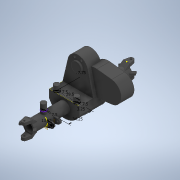
# Autodesk Inventor part: RCT-P004_front_rear_axle_simplified
Saved by Autodesk Inventor 2020 (Build 240168000, 168)
## iProperties
Created: 2019-11-14
Part Number: RCT-P004_front_rear_axle_simplified
Material: Generic
Document SubType Name: Modeling
Designer: maste
Density: 1 g/cm^3
Appearance: Generic
Author: maste
Autodesk Inventor part; units mm, degrees
ref_plane "YZ Plane" through (0, 0, 0) normal (1, 0, 0) x (0, 1, 0)
ref_plane "XZ Plane" through (0, 0, 0) normal (0, 1, 0) x (-1, 0, 0)
ref_plane "XY Plane" through (0, 0, 0) normal (0, 0, 1) x (1, 0, 0)
sketch "Sketch1" plane through (0, 0, 0) normal (0, 0, 1) x (1, 0, 0)
  circle A0 centre (0, 0) radius 8
  circle A1 centre (0, 0) radius 6
  dimension "d0" = 16
  dimension "d1" = 12
  constraints: 2 centre point, 2 coincident
  measures "d0" diameter of A0
  measures "d1" diameter of A1
extrude "Extrusion1" add sketch "Sketch1" along normal blind 145
sketch "Sketch2" plane through (0, 0, 145) normal (0, 0, 1) x (1, 0, 0)
  line L0 (-5, 11.75) -> (5, 11.75)
  line L1 (5, 11.75) -> (5, -11.75) construction
  line L2 (5, -11.75) -> (-5, -11.75)
  line L3 (-5, -11.75) -> (-5, 11.75) construction
  line L4 (-5, 7.75) -> (5, 7.75)
  line L5 (-5, -7.75) -> (5, -7.75)
  line L6 (-5, 11.75) -> (-5, 7.75)
  line L7 (5, 11.75) -> (5, 7.75)
  line L8 (-5, -7.75) -> (-5, -11.75)
  line L9 (5, -7.75) -> (5, -11.75)
  point P0 (0, 0)
  dimension "d4" = 23.5
  dimension "d5" = 10
  dimension "d6" = 5
  dimension "d7" = 11.75
  dimension "d8" = 10
  dimension "d9" = 4
  dimension "d10" = 0
  dimension "d11" = 4
  dimension "d12" = 10
  dimension "d13" = 0
  constraints: 20 end point, 3 horizontal, 2 parallel, 1 perpendicular
  measures "d4" distance of L0.end L1.end
  measures "d5" distance of L0.start L0.end
  measures "d6" distance from line of L3 point (0, 0)
  measures "d7" distance from line of L0 point (0, 0)
  measures "d8" distance of L4.start L4.end
  measures "d9" distance between parallel lines of L4 L0
  measures "d10" distance from line of L3 L4.start
  measures "d11" distance between parallel lines of L2 L5
  measures "d12" distance of L5.start L5.end
  measures "d13" distance from line of L1 L5.end
extrude "Extrusion2" add sketch "Sketch2" along normal blind 10
sketch "Sketch3" plane through (-5, 11.75, 145) normal (0, 1, 0) x (1, 0, 0)
  circle A0 centre (5, -6.45) radius 1.25
  line L0 (6.9843, 0) -> (13, 0) projected
  line L1 (11, 0) -> (-1, 0) projected
  circle A1 centre (5, -6.45) radius 3.55
  line L2 (0, 0) -> (0, -10) projected
  line L3 (10, -10) -> (0, -10) projected
  line L4 (10, 0) -> (10, -10) projected
  line L5 (10, 0) -> (8.4725, -7.1879)
  line L6 (0, 0) -> (0, -10) projected
  line L7 (0, 0) -> (1.5275, -7.1879)
  line L8 (0, 0) -> (0, -10)
  line L9 (0, -10) -> (10, -10) projected
  line L10 (0, -10) -> (10, -10)
  line L11 (0, 0) -> (10, 0) projected
  line L12 (10, -10) -> (10, 0)
  point P0 (5, 145)
  point P1 (5, -10)
  dimension "d16" = 2.5
  dimension "d21" = 7.1
  dimension "d22" = 5
  dimension "d23" = 3.55
  constraints: 10 end point, 2 centre point, 2 point on circle, 2 tangent, 1 coincident, 1 collinear, 1 perpendicular, 1 vertical
  measures "d16" diameter of A0
  measures "d21" diameter of A1
  measures "d22" distance from line of L2 A0.centre
  measures "d23" distance from line of L3 A0.centre
extrude "Extrusion3" cut sketch "Sketch3" against normal through all contours A0 | L4 L3 A1 L5 | L7 A1 L3 L2
sketch "Sketch4" plane through (0, 0, 0) normal (0, 0, -1) x (-1, 0, 0)
  line L0 (5, -11.75) -> (-5, -11.75) projected
  line L1 (-5, 11.75) -> (5, 11.75) projected
  line L2 (-5, -11.75) -> (5, -11.75)
  line L3 (5, 11.75) -> (-5, 11.75)
  line L4 (-1.9843, 7.75) -> (-5, 7.75) projected
  line L5 (5, 7.75) -> (1.9843, 7.75) projected
  line L6 (-5, 7.75) -> (5, 7.75)
  line L7 (-5, -7.75) -> (-1.9843, -7.75) projected
  line L8 (1.9843, -7.75) -> (5, -7.75) projected
  line L9 (-5, -7.75) -> (5, -7.75)
  line L10 (-5, 11.75) -> (-5, 7.75)
  line L11 (-5, -7.75) -> (-5, -11.75)
  line L12 (5, -11.75) -> (5, -7.75)
  line L13 (5, 7.75) -> (5, 11.75)
  point P0 (0, 0)
  point P1 (-1.9843, -7.75)
  point P2 (1.9843, 7.75)
  constraints: 16 end point, 5 parallel, 2 horizontal, 2 perpendicular, 1 collinear
extrude "Extrusion4" add sketch "Sketch4" along normal blind 10
sketch "Sketch5" plane through (-5, 11.75, 0) normal (0, 1, 0) x (1, 0, 0)
  circle A0 centre (5, 6.45) radius 1.25
  circle A1 centre (5, 6.45) radius 3.55
  line L0 (0, 0) -> (0, 10) projected
  line L1 (0, 10) -> (10, 10) projected
  line L2 (0, 0) -> (0, 10) projected
  line L3 (0, 0) -> (1.5275, 7.1879)
  line L4 (10, 0) -> (10, 10) projected
  line L5 (10, 0) -> (8.4725, 7.1879)
  line L6 (10, 10) -> (0, 10) projected
  line L7 (10, 0) -> (10, 10)
  line L8 (10, 10) -> (0, 10)
  line L9 (0, 10) -> (0, 0)
  point P0 (5, 0)
  point P1 (5, 10)
  dimension "d28" = 2.5
  dimension "d29" = 7.1
  dimension "d30" = 5
  dimension "d31" = 3.55
  constraints: 10 end point, 3 perpendicular, 2 centre point, 2 point on circle, 2 tangent, 1 coincident
  measures "d28" diameter of A0
  measures "d29" diameter of A1
  measures "d30" distance from line of L0 A0.centre
  measures "d31" distance from line of L1 A0.centre
extrude "Extrusion5" cut sketch "Sketch5" against normal through all contours A0 | A1 L1 L4 L5 | L3 L0 L1 A1
ref_plane "Work Plane1" through (5, 7.75, 145) normal (-1, 0, 0) x (0, 1, 0)
sketch "Sketch6" plane through (5, 7.75, 145) normal (-1, 0, 0) x (0, 1, 0)
  line L0 (4, 0) -> (0, 0) projected
  line L1 (4, 0) -> (-1, 0)
  line L2 (-1, 0) -> (-1, 7) construction
  line L3 (-1, 7) -> (4, 7) construction
  line L4 (4, 7) -> (4, 0) construction
  line L5 (4, 0) -> (-1, 7)
  line L6 (-19.5, 0) -> (-14.5, 0)
  line L7 (-14.5, 0) -> (-14.5, 7) construction
  line L8 (-14.5, 7) -> (-19.5, 7) construction
  line L9 (-19.5, 7) -> (-19.5, 0) construction
  line L10 (-14.5, 7) -> (-19.5, 0)
  line L11 (4, 145) -> (0, 145) projected
  line L12 (4, 145) -> (-1, 145)
  line L13 (-1, 145) -> (-1, 138) construction
  line L14 (-1, 138) -> (4, 138) construction
  line L15 (4, 138) -> (4, 145) construction
  line L16 (4, 145) -> (-1, 138)
  line L17 (-15.5, 145) -> (-19.5, 145) projected
  line L18 (-19.5, 145) -> (-14.5, 145)
  line L19 (-14.5, 145) -> (-14.5, 138) construction
  line L20 (-14.5, 138) -> (-19.5, 138) construction
  line L21 (-19.5, 138) -> (-19.5, 145) construction
  line L22 (-19.5, 145) -> (-14.5, 138)
  line L23 (-15.5, 0) -> (0, 0) projected
  line L24 (-1, 7) -> (-1.5, 7)
  line L25 (-1.5, 7) -> (-1.5, 0)
  line L26 (-1.5, 0) -> (-1, 0)
  line L27 (-1, 0) -> (-1, 7) construction
  line L28 (-14.5, 7) -> (-14, 7)
  line L29 (-14, 7) -> (-14, 0)
  line L30 (-14, 0) -> (-14.5, 0)
  line L31 (-14.5, 0) -> (-14.5, 7) construction
  line L32 (-15.5, 145) -> (0, 145) projected
  line L33 (-1, 138) -> (-1.5, 138)
  line L34 (-1.5, 138) -> (-1.5, 145)
  line L35 (-1.5, 145) -> (-1, 145)
  line L36 (-1, 145) -> (-1, 138) construction
  line L37 (-14.5, 138) -> (-14, 138)
  line L38 (-14, 138) -> (-14, 145)
  line L39 (-14, 145) -> (-14.5, 145)
  line L40 (-14.5, 145) -> (-14.5, 138) construction
  point P0 (-7.75, 145)
  point P1 (0, 145)
  point P2 (0, 0)
  dimension "d35" = 5
  dimension "d36" = 7
  dimension "d37" = 5
  dimension "d38" = 7
  dimension "d39" = 5
  dimension "d40" = 7
  dimension "d41" = 5
  dimension "d42" = 7
  dimension "d45" = 0.5
  dimension "d46" = 0.5
  dimension "d47" = 0.5
  dimension "d48" = 0.5
  constraints: 72 end point, 16 parallel, 8 horizontal, 8 perpendicular, 2 point on line, 3 other
  measures "d35" distance of L2.end L3.end
  measures "d36" distance of L3.end L0.start
  measures "d37" distance of L8.end L7.end
  measures "d38" distance of L6.end L7.end
  measures "d39" distance of L14.end L13.end
  measures "d40" distance of L14.end L11.start
  measures "d41" distance of L19.end L20.end
  measures "d42" distance of L18.end L19.end
  measures "d45" distance of L26.end L25.end
  measures "d46" distance of L29.end L30.end
  measures "d47" distance of L34.end L35.end
  measures "d48" distance of L39.end L38.end
extrude "Extrusion7" add sketch "Sketch6" along normal blind 10
sketch "Sketch7" plane through (0, 0, 0) normal (0, 1, 0) x (-1, 0, 0)
  line L0 (12.5, 149.25) -> (-12.5, 149.25) construction
  line L1 (-12.5, 149.25) -> (-12.5, -4.25) construction
  line L2 (-12.5, -4.25) -> (12.5, -4.25) construction
  line L3 (12.5, -4.25) -> (12.5, 149.25) construction
  line L4 (0, -74.8115) -> (0, 193.3019) projected
  arc A0 (3.4725, 152.1879) -> (-3.4725, 152.1879) centre (0, 151.45) ccw projected
  line L5 (17.5, 0) -> (-17.5, 0) projected
  line L6 (12.5, -4.25) -> (10.25, -4.25) construction
  line L7 (10.25, -4.25) -> (10.25, -0.5) construction
  line L8 (10.25, -0.5) -> (12.5, -0.5) construction
  line L9 (12.5, -0.5) -> (12.5, -4.25) construction
  line L10 (-12.5, -4.25) -> (-10.25, -4.25) construction
  line L11 (-10.25, -4.25) -> (-10.25, -0.5) construction
  line L12 (-10.25, -0.5) -> (-12.5, -0.5) construction
  line L13 (-12.5, -0.5) -> (-12.5, -4.25) construction
  line L14 (12.5, 149.25) -> (10.25, 149.25) construction
  line L15 (10.25, 149.25) -> (10.25, 145.5) construction
  line L16 (10.25, 145.5) -> (12.5, 145.5) construction
  line L17 (12.5, 145.5) -> (12.5, 149.25) construction
  line L18 (-12.5, 149.25) -> (-10.25, 149.25) construction
  line L19 (-10.25, 149.25) -> (-10.25, 145.5) construction
  line L20 (-10.25, 145.5) -> (-12.5, 145.5) construction
  line L21 (-12.5, 145.5) -> (-12.5, 149.25) construction
  line L22 (-10.3818, -4.0303) -> (-12.4197, -0.6339)
  line L23 (-10.0689, -4.0689) -> (-6, 0)
  line L24 (-6, 145) -> (-6, 0) projected
  line L25 (-12.3896, -0.3896) -> (-6, 6)
  line L26 (-6, 0) -> (-6, 6)
  line L27 (10.3818, -4.0303) -> (12.4197, -0.6339)
  line L28 (10.0689, -4.0689) -> (6, 0)
  line L29 (6, 145) -> (6, 0) projected
  line L30 (12.3896, -0.3896) -> (6, 6)
  line L31 (6, 0) -> (6, 6)
  line L32 (8, 0) -> (4.9937, 0) projected
  line L33 (12.4197, 145.6339) -> (10.3818, 149.0303)
  line L34 (6, 145) -> (10.0689, 149.0689)
  line L35 (12.3896, 145.3896) -> (6, 139)
  line L36 (6, 139) -> (6, 145)
  line L37 (-12.4197, 145.6339) -> (-10.3818, 149.0303)
  line L38 (-10.0689, 149.0689) -> (-6, 145)
  line L39 (-12.3896, 145.3896) -> (-6, 139)
  line L40 (-6, 145) -> (-6, 139)
  arc A1 (10.0689, -4.0689) -> (10.3818, -4.0303) centre (10.2103, -3.9274) ccw
  arc A2 (12.4197, -0.6339) -> (12.3896, -0.3896) centre (12.2482, -0.531) ccw
  arc A3 (-10.3818, -4.0303) -> (-10.0689, -4.0689) centre (-10.2103, -3.9274) ccw
  arc A4 (-12.3896, -0.3896) -> (-12.4197, -0.6339) centre (-12.2482, -0.531) ccw
  arc A5 (12.3896, 145.3896) -> (12.4197, 145.6339) centre (12.2482, 145.531) ccw
  arc A6 (10.3818, 149.0303) -> (10.0689, 149.0689) centre (10.2103, 148.9274) ccw
  arc A7 (-12.4197, 145.6339) -> (-12.3896, 145.3896) centre (-12.2482, 145.531) ccw
  arc A8 (-10.0689, 149.0689) -> (-10.3818, 149.0303) centre (-10.2103, 148.9274) ccw
  point P0 (0, 0)
  dimension "d51" = 25
  dimension "d52" = 153.5
  dimension "d53" = 12.5
  dimension "d55" = 4.25
  dimension "d56" = 3.75
  dimension "d57" = 2.25
  dimension "d58" = 3.75
  dimension "d59" = 2.25
  dimension "d60" = 3.75
  dimension "d61" = 2.25
  dimension "d62" = 3.75
  dimension "d63" = 2.25
  dimension "d64" = 0.2
  constraints: 72 end point, 22 point on line, 16 point on circle, 16 tangent, 14 parallel, 8 centre point, 7 equal radius, 6 perpendicular, 5 horizontal, 2 collinear, 1 vertical, 3 other
  measures "d51" distance of L0.start L0.end
  measures "d52" distance of L2.end L0.start
  measures "d53" distance between parallel lines of L4 L3
  measures "d55" distance of the line from the sketch origin of L2
  measures "d56" distance of L6.end L7.end
  measures "d57" distance of L7.end L8.end
  measures "d58" distance of L10.end L11.end
  measures "d59" distance of L11.end L12.end
  measures "d60" distance of L14.end L15.end
  measures "d61" distance of L15.end L16.end
  measures "d62" distance of L18.end L19.end
  measures "d63" distance of L19.end L20.end
  measures "d64" radius of A1
extrude "Extrusion8" add sketch "Sketch7" along normal blind 2.5
ref_plane "Work Plane2" through (0, 0, 125.5) normal (0, 0, 1) x (1, 0, 0)
sketch "Sketch8" plane through (0, 0, 125.5) normal (0, 0, 1) x (1, 0, 0)
  line L0 (0, 0) -> (13.85, 0) construction
  line L1 (10.3818, 0) -> (12.4197, 0) construction
  circle A0 centre (13.85, 0) radius 1.25
  arc A1 (14.8366, -3.3581) -> (13.85, 3.5) centre (13.85, 0) ccw
  arc A2 (4.9937, -6.25) -> (8, 0) centre (0, 0) ccw projected
  line L2 (4.9937, -6.25) -> (14.8366, -3.3581)
  line L3 (13.85, 3.5) -> (7.1937, 3.5)
  line L4 (4.9937, -6.25) -> (7.1937, 3.5)
  arc A3 (7.5993, 2.5) -> (4.9937, 6.25) centre (0, 0) ccw projected
  dimension "d68" = 13.85
  dimension "d69" = 2.5
  dimension "d70" = 7
  constraints: 8 end point, 3 point on circle, 2 centre point, 2 coincident, 2 tangent, 1 collinear, 1 horizontal
  measures "d68" distance of L0.start L0.end
  measures "d69" diameter of A0
  measures "d70" diameter of A1
extrude "Extrusion9" add sketch "Sketch8" against normal blind 2.5
ref_plane "Work Plane3" through (0, 0, 116) normal (0, 0, 1) x (1, 0, 0)
sketch "Sketch9" plane through (0, 0, 116) normal (0, 0, 1) x (1, 0, 0)
  line L0 (0, 0) -> (13.85, 0) construction
  circle A0 centre (13.85, 0) radius 1.25
  arc A1 (14.8366, -3.3581) -> (13.85, 3.5) centre (13.85, 0) ccw
  line L1 (4.9937, -6.25) -> (14.8366, -3.3581)
  line L2 (13.85, 3.5) -> (7.1937, 3.5)
  line L3 (4.9937, -6.25) -> (7.1937, 3.5)
  dimension "d74" = 13.85
  dimension "d75" = 2.5
  dimension "d76" = 7
  constraints: 8 end point, 2 centre point, 2 coincident, 2 point on circle, 2 tangent, 1 horizontal
  measures "d74" distance of L0.start L0.end
  measures "d75" diameter of A0
  measures "d76" diameter of A1
extrude "Extrusion10" add sketch "Sketch9" against normal blind 2.5
ref_plane "Work Plane4" through (0, 0, 31.5) normal (0, 0, 1) x (1, 0, 0)
sketch "Sketch10" plane through (0, 0, 31.5) normal (0, 0, 1) x (1, 0, 0)
  line L0 (0, 0) -> (13.85, 0) construction
  circle A0 centre (13.85, 0) radius 1.25
  arc A1 (14.8366, -3.3581) -> (13.85, 3.5) centre (13.85, 0) ccw
  line L1 (4.9937, -6.25) -> (14.8366, -3.3581)
  line L2 (13.85, 3.5) -> (7.1937, 3.5)
  line L3 (4.9937, -6.25) -> (7.1937, 3.5)
  dimension "d80" = 13.85
  dimension "d81" = 2.5
  dimension "d82" = 7
  constraints: 8 end point, 2 centre point, 2 coincident, 2 point on circle, 2 tangent, 1 horizontal
  measures "d80" distance of L0.start L0.end
  measures "d81" diameter of A0
  measures "d82" diameter of A1
extrude "Extrusion11" add sketch "Sketch10" against normal blind 2.5
ref_plane "Work Plane5" through (0, 0, 22) normal (0, 0, 1) x (1, 0, 0)
sketch "Sketch11" plane through (0, 0, 22) normal (0, 0, 1) x (1, 0, 0)
  line L0 (0, 0) -> (13.85, 0) construction
  circle A0 centre (13.85, 0) radius 1.25
  arc A1 (14.8366, -3.3581) -> (13.85, 3.5) centre (13.85, 0) ccw
  line L1 (4.9937, -6.25) -> (14.8366, -3.3581)
  line L2 (13.85, 3.5) -> (7.1937, 3.5)
  line L3 (4.9937, -6.25) -> (7.1937, 3.5)
  dimension "d86" = 13.85
  dimension "d87" = 2.5
  dimension "d88" = 7
  constraints: 8 end point, 2 centre point, 2 coincident, 2 point on circle, 2 tangent, 1 horizontal
  measures "d86" distance of L0.start L0.end
  measures "d87" diameter of A0
  measures "d88" diameter of A1
extrude "Extrusion12" add sketch "Sketch11" against normal blind 2.5
sketch "Sketch12" plane through (0, 0, 0) normal (0, 1, 0) x (-1, 0, 0)
  line L0 (22.5, 53) -> (-22.5, 53)
  line L1 (-22.5, 53) -> (-22.5, 92)
  line L2 (-22.5, 92) -> (22.5, 92)
  line L3 (22.5, 92) -> (22.5, 53)
  line L4 (25.5719, 0) -> (-37.4281, 0) projected
  line L5 (0, -43) -> (0, 188) projected
  point P0 (0, 0)
  dimension "d91" = 39
  dimension "d92" = 45
  dimension "d93" = 92
  dimension "d94" = 22.5
  constraints: 8 end point, 2 parallel, 1 horizontal, 1 perpendicular
  measures "d91" distance of L0.end L1.end
  measures "d92" distance of L0.start L0.end
  measures "d93" distance between parallel lines of L4 L2
  measures "d94" distance between parallel lines of L5 L1
extrude "Extrusion13" add sketch "Sketch12" along normal blind 11.75
sketch "Sketch13" plane through (0, 11.75, 0) normal (0, 1, 0) x (1, 0, 0)
  line L0 (-14.75, -88.75) -> (14.75, -88.75) construction
  line L1 (-22.5, -92) -> (22.5, -92) construction
  line L2 (-22.5, -53) -> (-22.5, -92) construction
  circle A0 centre (-14.75, -88.75) radius 3.75
  circle A1 centre (14.75, -88.75) radius 3.75
  circle A2 centre (0, -123) radius 3.75
  point P0 (0, 0)
  dimension "d97" = 29.5
  dimension "d98" = 3.25
  dimension "d99" = 7.75
  dimension "d100" = 7.5
  dimension "d101" = 7.5
  dimension "d109" = 7.5
  dimension "d110" = 34.25
  constraints: 3 centre point, 2 coincident, 2 end point, 1 horizontal
  measures "d97" distance of L0.start L0.end
  measures "d98" distance between parallel lines of L1 L0
  measures "d99" distance from line of L2 L0.start
  measures "d100" diameter of A0
  measures "d101" diameter of A1
  measures "d109" diameter of A2
  measures "d110" vertical distance of A2.centre L0.end
extrude "Extrusion14" add sketch "Sketch13" along normal blind 8.3 contours A0 | A1
extrude "Extrusion16" add sketch "Sketch13" along normal blind 9.3 and the other way blind 5 contours A2
sketch "Sketch14" plane through (8, 0, 92) normal (0, 0, 1) x (1, 0, 0)
  line L0 (-8, 0) -> (-8, -14.8) construction
  line L1 (-30.5, 0) -> (-30.5, 11.75) construction
  line L2 (14.5, 0) -> (14.5, 11.75) construction
  arc A0 (-30.5, 0) -> (14.5, 0) centre (-8, 9.703) ccw
  line L3 (-30.5, 0) -> (14.5, 0)
  dimension "d115" = 14.8
  constraints: 4 end point, 3 point on circle, 1 centre point, 1 horizontal, 1 vertical
  measures "d115" distance of L0.start L0.end
extrude "Extrusion17" add sketch "Sketch14" against normal blind 39
sketch "Sketch15" plane through (22.5, 11.75, 53) normal (0, 0, -1) x (-1, 0, 0)
  line L0 (17.5, 0) -> (27.5, 0) construction
  line L1 (22.5, 0) -> (22.5, 44.8) construction
  arc A0 (37.0935, 33.2683) -> (7.9065, 33.2683) centre (22.5, 29.8) ccw
  line L2 (0, 0) -> (45, 0) projected
  line L3 (45, 0) -> (37.0935, 33.2683)
  line L4 (0, 0) -> (7.9065, 33.2683)
  line L5 (0, 0) -> (45, 0)
  point P0 (22.5, -11.75)
  dimension "d118" = 44.8
  dimension "d119" = 30
  dimension "d120" = 15
  constraints: 8 end point, 2 point on circle, 2 tangent, 1 centre point, 1 collinear, 1 midpoint, 1 point on line, 1 vertical
  measures "d118" distance of L1.start L1.end
  measures "d119" diameter of A0
  measures "d120" distance of L1.end A0.centre
extrude "Extrusion18" add sketch "Sketch15" against normal blind 19
sketch "Sketch16" plane through (22.5, 11.75, 72) normal (0, 0, 1) x (1, 0, 0)
  arc A0 (-7.9065, 33.2683) -> (-37.0935, 33.2683) centre (-22.5, 29.8) ccw projected
  circle A1 centre (-22.5, 29.8) radius 7.5
  point P0 (-22.5, -11.75)
  dimension "d123" = 15
  constraints: 1 centre point, 1 coincident
  measures "d123" diameter of A1
extrude "Extrusion19" add sketch "Sketch16" along normal blind 2.5
sketch "Sketch17" plane through (22.5, 11.75, 72) normal (0, 0, 1) x (1, 0, 0)
  circle A0 centre (-22.5, 29.8) radius 7.5 construction
  line L0 (-22.5, 29.8) -> (-17.5, 29.8) construction
  line L1 (-17.5, 29.8) -> (-17.5, 39.8) construction
  line L2 (-17.5, 39.8) -> (-22.5, 39.8) construction
  line L3 (-22.5, 39.8) -> (-22.5, 29.8) construction
  line L4 (-22.5, 29.8) -> (-27.5, 29.8) construction
  line L5 (-27.5, 29.8) -> (-27.5, 39.8) construction
  line L6 (-27.5, 39.8) -> (-22.5, 39.8) construction
  line L7 (-22.5, 39.8) -> (-22.5, 29.8) construction
  circle A1 centre (-17.5, 39.8) radius 1.5
  circle A2 centre (-27.5, 39.8) radius 1.5
  point P0 (-22.5, -11.75)
  dimension "d126" = 5
  dimension "d127" = 10
  dimension "d128" = 5
  dimension "d129" = 10
  dimension "d130" = 3
  dimension "d131" = 3
  constraints: 16 end point, 4 parallel, 2 centre point, 2 coincident, 2 horizontal, 2 perpendicular
  measures "d126" distance of L2.end L1.end
  measures "d127" distance of L0.end L1.end
  measures "d128" distance of L5.end L6.end
  measures "d129" distance of L4.end L5.end
  measures "d130" diameter of A1
  measures "d131" diameter of A2
extrude "Extrusion20" cut sketch "Sketch17" against normal blind 3
sketch "Sketch18" plane through (0, 9.703, 53) normal (0, 0, -1) x (-1, 0, 0)
  arc A0 (-44.9559, 35.2447) -> (-44.9559, 3.4492) centre (-43.15, 19.347) ccw
  arc A1 (-23.088, 0.9652) -> (-23.088, 37.7287) centre (-21, 19.347) ccw
  line L0 (-44.9559, 35.2447) -> (-23.088, 37.7287)
  line L1 (-44.9559, 3.4492) -> (-23.088, 0.9652)
  point P0 (0, -9.703)
  point P1 (-34.022, 6.2062)
  point P2 (-34.022, 32.4877)
  dimension "d134" = 32
  dimension "d135" = 29.05
  dimension "d136" = 43.15
  dimension "d137" = 37
  dimension "d138" = 29.05
  dimension "d139" = 21
  constraints: 4 end point, 4 point on circle, 4 tangent, 2 centre point
  measures "d134" diameter of A0
  measures "d135" vertical distance of point (0, -9.703) A0.centre
  measures "d136" horizontal distance of point (0, -9.703) A0.centre
  measures "d137" diameter of A1
  measures "d138" vertical distance of point (0, -9.703) A1.centre
  measures "d139" horizontal distance of point (0, -9.703) A1.centre
extrude "Extrusion21" add sketch "Sketch18" along normal blind 5 and the other way blind 14
body "Solid1"
